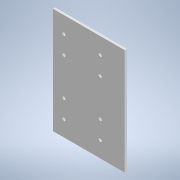
# Autodesk Inventor part: Part3
Saved by Autodesk Inventor 2020.2 (Build 242310000, 310)
## iProperties
Created: 2022-11-14
Part Number: Part3
Material: 一般
Document SubType Name: Modeling
Designer: Administrator
Density: 1 g/cm^3
Appearance: 既定
Author: Administrator
Autodesk Inventor part; units mm, degrees
ref_plane "YZ Plane" through (0, 0, 0) normal (1, 0, 0) x (0, 1, 0)
ref_plane "XZ Plane" through (0, 0, 0) normal (0, 1, 0) x (-1, 0, 0)
ref_plane "XY Plane" through (0, 0, 0) normal (0, 0, 1) x (1, 0, 0)
sketch "スケッチ1" plane through (0, 0, 0) normal (1, 0, 0) x (0, 1, 0)
  point P0 (0, 0)
sketch "スケッチ2" plane through (0, 0, 0) normal (0, 0, 1) x (1, 0, 0)
  line L0 (-24.05, -44.1) -> (-24.05, -30.9) projected
  line L1 (-2, -44.1) -> (-24.05, -44.1) projected
  line L2 (-2, -0.9) -> (-2, -44.1) projected
  line L3 (-56.5, -0.9) -> (-2, -0.9) projected
  line L4 (-56.5, -0.9) -> (-56.5, -44.1) projected
  line L5 (-37.25, -44.1) -> (-56.5, -44.1) projected
  line L6 (-37.25, -44.1) -> (-37.25, -30.9) projected
  line L7 (-37.25, -30.9) -> (-24.05, -30.9) projected
  circle A0 centre (-19.75, -14.5) radius 1.35 projected
  circle A1 centre (-51.75, -30.5) radius 1.35 projected
  circle A2 centre (-51.75, -14.5) radius 1.35 projected
  circle A3 centre (-19.75, -30.5) radius 1.35 projected
  line L8 (-24.05, -63.1) -> (-24.05, -49.9) projected
  line L9 (-24.05, -63.1) -> (-37.25, -63.1) projected
  line L10 (-37.25, -63.1) -> (-37.25, -49.9) projected
  line L11 (-56.5, -49.9) -> (-37.25, -49.9) projected
  line L12 (-56.5, -93.1) -> (-56.5, -49.9) projected
  line L13 (-2, -93.1) -> (-56.5, -93.1) projected
  line L14 (-2, -93.1) -> (-2, -49.9) projected
  line L15 (-24.05, -49.9) -> (-2, -49.9) projected
  circle A4 centre (-19.75, -79.5) radius 1.35 projected
  circle A5 centre (-51.75, -63.5) radius 1.35 projected
  circle A6 centre (-51.75, -79.5) radius 1.35 projected
  circle A7 centre (-19.75, -63.5) radius 1.35 projected
  line L16 (0, 0) -> (0, -93.5) projected
  line L17 (0, -93.5) -> (2, -93.5) projected
  line L18 (2, 0) -> (2, -93.5) projected
  line L19 (0, 0) -> (2, 0) projected
  line L20 (2, 0) -> (-61.4413, 0)
  line L21 (-61.4413, 0) -> (-61.4413, -93.5)
  line L22 (-61.4413, -93.5) -> (2, -93.5)
  line L23 (2, -93.5) -> (2, 0)
  constraints: 8 end point, 2 parallel, 1 horizontal, 1 perpendicular
extrude "押し出し1" add sketch "スケッチ2" along normal blind 2 contours L0 L7 L6 L5 L4 L3 L2 L1 | L8 L15 L14 L13 L12 L11 L10 L9 | L19 L18 L17 L16 | L16 L22 L21 L20
